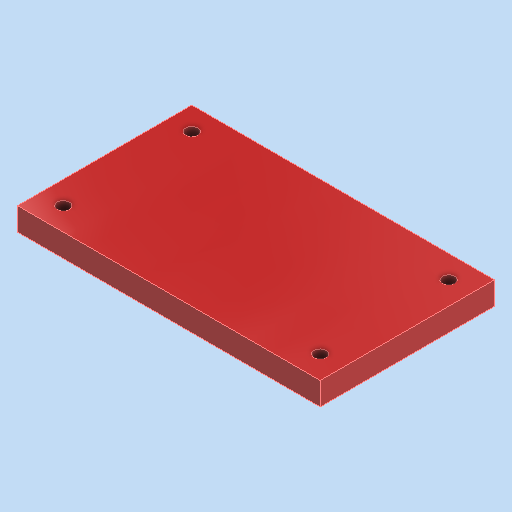
# Autodesk Inventor part: драйвер двигателя
Saved by Autodesk Inventor 2025 (Build 290162000, 162)
## iProperties
Created: 2025-03-03
Part Number: драйвер двигателя
Material: Типовые
Document SubType Name: Modeling
Designer: volko
Density: 1 g/cm^3
Appearance: По умолчанию
Author: volko
Autodesk Inventor part; units mm, degrees
ref_plane "YZ Plane" through (0, 0, 0) normal (1, 0, 0) x (0, 1, 0)
ref_plane "XZ Plane" through (0, 0, 0) normal (0, 1, 0) x (-1, 0, 0)
ref_plane "XY Plane" through (0, 0, 0) normal (0, 0, 1) x (1, 0, 0)
sketch "Эскиз1" plane through (0, 0, 0) normal (0, 1, 0) x (-1, 0, 0)
  line L0 (33, -19) -> (-33, -19)
  line L1 (-33, -19) -> (-33, 19)
  line L2 (-33, 19) -> (33, 19)
  line L3 (33, 19) -> (33, -19)
  line L4 (0, -26.6) -> (0, 26.6) projected
  line L5 (46.2, 0) -> (-46.2, 0) projected
  circle A0 centre (28, -14) radius 1.35
  circle A1 centre (28, 14) radius 1.35
  circle A2 centre (-28, -14) radius 1.35
  circle A3 centre (-28, 14) radius 1.35
  point P0 (0, 0)
  dimension "d0" = 66
  dimension "d1" = 38
  dimension "d11" = 2.7
  dimension "d12" = 5
  dimension "d13" = 5
  constraints: 8 end point, 4 centre point, 3 symmetric about line, 2 parallel, 1 horizontal, 1 perpendicular, 5 other
  measures "d0" distance of L0.start L0.end
  measures "d1" distance of L0.end L1.end
  measures "d11" diameter of A0
  measures "d12" distance from line of A0.centre L0
  measures "d13" distance from line of A0.centre L3
extrude "Выдавливание1" add sketch "Эскиз1" along normal blind 5
